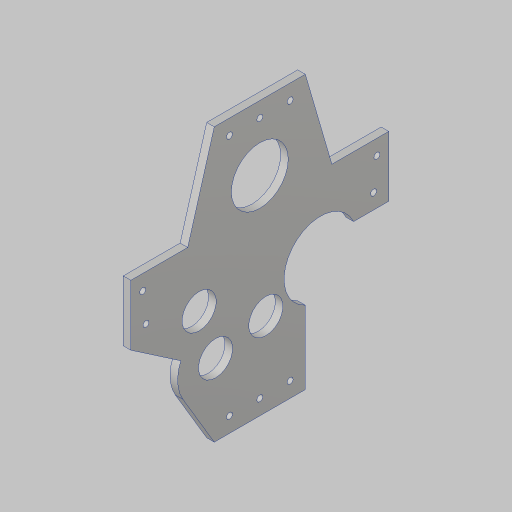
# Autodesk Inventor part: EL2-CGB-003
Saved by Autodesk Inventor 2023.5 (Build 275446000, 446)
## iProperties
Created: 2025-01-19
Part Number: EL2-CGB-003
Material: Aluminum 6061
Document SubType Name: Modeling
Designer: mavericks
Density: 2.7 g/cm^3
Appearance: Aluminum - Flat
Author: mavericks
Autodesk Inventor part; units mm, degrees
ref_plane "YZ Plane" through (0, 0, 0) normal (1, 0, 0) x (0, 1, 0)
ref_plane "XZ Plane" through (0, 0, 0) normal (0, 1, 0) x (-1, 0, 0)
ref_plane "XY Plane" through (0, 0, 0) normal (0, 0, 1) x (1, 0, 0)
sketch "Sketch1" plane through (0, 0, 0) normal (1, 0, 0) x (0, 1, 0)
  line L0 (114.3, 107.95) -> (-114.3, 107.95) construction
  line L1 (-114.3, 107.95) -> (-114.3, 82.55) construction
  line L2 (-114.3, 82.55) -> (114.3, 82.55) construction
  line L3 (114.3, 82.55) -> (114.3, 107.95) construction
  line L4 (-44.45, 128.7526) -> (-69.85, 128.7526) construction
  line L5 (-69.85, 128.7526) -> (-69.85, 79.4258) construction
  line L6 (-69.85, 79.4258) -> (-44.45, 79.4258) construction
  line L7 (-44.45, 79.4258) -> (-44.45, 128.7526) construction
  line L8 (69.85, 128.7526) -> (44.45, 128.7526) construction
  line L9 (44.45, 128.7526) -> (44.45, 79.4258) construction
  line L10 (44.45, 79.4258) -> (69.85, 79.4258) construction
  line L11 (69.85, 79.4258) -> (69.85, 128.7526) construction
  line L12 (44.45, 104.0892) -> (-44.45, 104.0892) construction
  line L13 (0, 0) -> (-27.2932, 0) construction
  line L14 (114.3, -107.95) -> (-114.3, -107.95) construction
  line L15 (-114.3, -107.95) -> (-114.3, -82.55) construction
  line L16 (-114.3, -82.55) -> (114.3, -82.55) construction
  line L17 (114.3, -82.55) -> (114.3, -107.95) construction
  line L18 (-44.45, -128.7526) -> (-69.85, -128.7526) construction
  line L19 (-69.85, -128.7526) -> (-69.85, -79.4258) construction
  line L20 (-69.85, -79.4258) -> (-44.45, -79.4258) construction
  line L21 (-44.45, -79.4258) -> (-44.45, -128.7526) construction
  line L22 (69.85, -128.7526) -> (44.45, -128.7526) construction
  line L23 (44.45, -128.7526) -> (44.45, -79.4258) construction
  line L24 (44.45, -79.4258) -> (69.85, -79.4258) construction
  line L25 (69.85, -79.4258) -> (69.85, -128.7526) construction
  line L26 (44.45, -104.0892) -> (-44.45, -104.0892) construction
  line L27 (114.3, 82.55) -> (88.9, 82.55) construction
  line L28 (88.9, 82.55) -> (88.9, -82.55) construction
  line L29 (88.9, -82.55) -> (114.3, -82.55) construction
  line L30 (114.3, -82.55) -> (114.3, 82.55) construction
  line L31 (-114.3, 82.55) -> (-88.9, 82.55) construction
  line L32 (-88.9, 82.55) -> (-88.9, -82.55) construction
  line L33 (-88.9, -82.55) -> (-114.3, -82.55) construction
  line L34 (-114.3, -82.55) -> (-114.3, 82.55) construction
  point P0 (0, 82.55)
  point P1 (0, 104.0892)
  point P2 (0, -82.55)
  point P3 (0, -104.0892)
  dimension "d0" = 228.6
  dimension "d1" = 25.4
  dimension "d2" = 82.55
  dimension "d3" = 25.4
  dimension "d4" = 49.3268
  dimension "d6" = 88.9
  dimension "d7" = 3.1242
  dimension "d8" = 25.4
  dimension "d9" = 25.4
  constraints: 70 end point, 16 symmetric about line, 12 parallel, 7 horizontal, 5 perpendicular, 4 midpoint, 2 vertical alignment, 1 horizontal alignment, 1 point on line
  measures "d0" distance of L2.end L1.end
  measures "d1" distance of L1.end L0.end
  measures "d2" vertical distance of L13.start L2.end
  measures "d3" distance of L6.end L5.end
  measures "d4" distance of L5.end L4.end
  measures "d6" distance of L4.start L8.end
  measures "d7" distance from line of L2 L6.end
  measures "d8" distance between parallel lines of L28 L30
  measures "d9" distance between parallel lines of L34 L32
sketch "Sketch2" plane through (0, 0, 0) normal (1, 0, 0) x (0, 1, 0)
  line L0 (-114.3, 107.95) -> (-114.3, 82.55) construction
  line L1 (44.45, 104.0892) -> (-44.45, 104.0892) construction
  line L2 (-114.3, 82.55) -> (114.3, 82.55) construction
  line L3 (114.3, 107.95) -> (-114.3, 107.95) construction
  line L4 (44.45, 79.4258) -> (69.85, 79.4258) construction
  line L5 (114.3, 82.55) -> (114.3, 107.95) construction
  line L6 (-69.85, 79.4258) -> (-44.45, 79.4258) construction
  line L7 (-44.45, 79.4258) -> (-44.45, 128.7526) construction
  line L8 (-69.85, 128.7526) -> (-69.85, 79.4258) construction
  line L9 (-44.45, 128.7526) -> (-69.85, 128.7526) construction
  line L10 (88.9, 82.55) -> (88.9, -82.55) construction
  line L11 (114.3, -82.55) -> (114.3, 82.55) construction
  line L12 (-114.3, -82.55) -> (114.3, -82.55) construction
  line L13 (114.3, -107.95) -> (-114.3, -107.95) construction
  line L14 (44.45, -104.0892) -> (-44.45, -104.0892) construction
  line L15 (-114.3, 82.55) -> (-88.9, 82.55) construction
  line L16 (-88.9, 82.55) -> (-88.9, -82.55) construction
  line L17 (-114.3, -82.55) -> (-114.3, 82.55) construction
  line L18 (-69.85, -79.4258) -> (-44.45, -79.4258) construction
  line L19 (-88.9, -82.55) -> (-114.3, -82.55) construction
  line L20 (-44.45, -79.4258) -> (-44.45, -128.7526) construction
  line L21 (-44.45, -128.7526) -> (-69.85, -128.7526) construction
  line L22 (-69.85, -128.7526) -> (-69.85, -79.4258) construction
  line L23 (-114.3, -107.95) -> (-114.3, -82.55) construction
  line L24 (44.45, -79.4258) -> (69.85, -79.4258) construction
  line L25 (44.45, -128.7526) -> (44.45, -79.4258) construction
  line L26 (88.9, -82.55) -> (114.3, -82.55) construction
  line L27 (69.85, -128.7526) -> (44.45, -128.7526) construction
  line L28 (69.85, -79.4258) -> (69.85, -128.7526) construction
  line L29 (114.3, -82.55) -> (114.3, -107.95) construction
  line L30 (69.85, 128.7526) -> (44.45, 128.7526) construction
  line L31 (44.45, 128.7526) -> (44.45, 79.4258) construction
  line L32 (69.85, 79.4258) -> (69.85, 128.7526) construction
  line L33 (114.3, 82.55) -> (88.9, 82.55) construction
  circle A0 centre (-25.4, -50.8) radius 7.62 construction
  circle A1 centre (-44.45, -5.08) radius 41.91 construction
  circle A2 centre (-44.45, -5.08) radius 11.43 construction
  circle A3 centre (-53.975, 37.0363) radius 31.75 construction
  circle A4 centre (-53.975, 37.0363) radius 15.24 construction
  circle A5 centre (-13.0473, 50.8) radius 27.94 construction
  circle A6 centre (-25.4, -50.8) radius 30.48 construction
  circle A7 centre (-25.4, -50.8) radius 10.16 construction
  circle A8 centre (-44.45, -5.08) radius 14.2875
  circle A9 centre (-53.975, 37.0363) radius 14.2875
  circle A10 centre (-13.0473, 50.8) radius 14.2875
  circle A11 centre (-13.0473, 50.8) radius 20.6375 construction
  circle A12 centre (-53.975, 37.0363) radius 20.6375 construction
  circle A13 centre (-44.45, -5.08) radius 20.6375 construction
  circle A14 centre (-25.4, -50.8) radius 17.4625 construction
  circle A15 centre (-25.4, -50.8) radius 25.4 construction
  line L34 (-41.275, -131.9276) -> (-41.275, -76.2508) construction
  line L35 (-41.275, -76.2508) -> (-73.025, -76.2508) construction
  line L36 (-73.025, -76.2508) -> (-73.025, -131.9276) construction
  line L37 (-73.025, -131.9276) -> (-41.275, -131.9276) construction
  line L38 (-114.3, -38.1) -> (-114.3, 38.1)
  line L39 (-114.3, 38.1) -> (-41.275, 38.1) construction
  line L40 (-41.275, 38.1) -> (-41.275, 104.0892) construction
  circle A16 centre (-25.4, -50.8) radius 30.48
  circle A17 centre (59.9086, 0) radius 23.8125
  circle A18 centre (59.9086, 0) radius 33.3375 construction
  line L41 (37.9487, 60.325) -> (114.3, 38.1)
  line L42 (114.3, 38.1) -> (114.3, -38.1)
  line L43 (114.3, -38.1) -> (37.9487, -60.325)
  line L44 (37.9487, -60.325) -> (37.9487, -107.95)
  line L45 (37.9487, -107.95) -> (-12.7, -107.95)
  line L46 (37.9487, 60.325) -> (37.9487, 107.95)
  line L47 (37.9487, 107.95) -> (-12.7, 107.95)
  circle A19 centre (-13.0473, 50.8) radius 20.6375 construction
  circle A20 centre (59.9086, 0) radius 57.277 construction
  line L48 (-12.7, 107.95) -> (-41.275, 66.1357)
  line L49 (-70.2044, 64.325) -> (-114.3, 38.1)
  arc A21 (-41.275, 66.1357) -> (-70.2044, 64.325) centre (-53.975, 37.0363) ccw
  line L50 (-53.1081, -38.1) -> (-114.3, -38.1)
  line L51 (-12.7, -78.5081) -> (-12.7, -107.95)
  point P0 (25.2487, 98.0186)
  point P1 (0, 95.25)
  point P2 (25.2487, -98.0186)
  point P3 (0, -95.25)
  point P4 (-25.4, -95.25)
  point P5 (-25.4, 95.25)
  point P6 (114.3, -95.25)
  point P7 (114.3, 95.25)
  point P8 (0, -82.55)
  point P9 (-101.6, 25.4)
  point P10 (-101.6, 0)
  point P11 (-101.6, -25.4)
  point P12 (-88.9, 0)
  point P13 (-101.6, 82.55)
  point P14 (-25.4, -25.4)
  point P15 (-25.4, -33.3375)
  point P16 (-47.397, -38.1)
  point P17 (-40.523, -42.0688)
  point P18 (-47.397, -63.5)
  point P19 (-40.523, -59.5312)
  point P20 (-25.4, -76.2)
  point P21 (-25.4, -68.2625)
  point P22 (-3.403, -63.5)
  point P23 (-10.277, -59.5313)
  point P24 (-3.403, -38.1)
  point P25 (-10.277, -42.0688)
  point P26 (44.45, 104.0892)
  point P27 (-41.275, -76.8195)
  point P28 (-114.3, 0)
  point P29 (-114.3, 0)
  point P30 (88.9, 0)
  point P31 (101.6, 25.4)
  point P32 (101.6, 0)
  point P33 (101.6, -25.4)
  point P34 (101.6, 82.55)
  point P35 (114.3, 0)
  dimension "d33" = 34.925
  dimension "d34" = 50.8
  dimension "d10" = 15.24
  dimension "d11" = 83.82
  dimension "d12" = 22.86
  dimension "d13" = 63.5
  dimension "d14" = 30.48
  dimension "d15" = 55.88
  dimension "d16" = 60.96
  dimension "d19" = 63.5
  dimension "d23" = 20.32
  dimension "d24" = 28.575
  dimension "d26" = 25.4
  dimension "d27" = 25.4
  dimension "d28" = 25.4
  dimension "d29" = 25.4
  dimension "d30" = 6.35
  dimension "d31" = 6.35
  dimension "d32" = 6.35
  dimension "d37" = 360
  dimension "d41" = 3.175
  dimension "d42" = 76.2
  dimension "d60" = 89.0513
  dimension "d63" = 31.75
  dimension "d64" = 44.45
  dimension "d66" = 34.925
  dimension "d67" = 31.75
  dimension "d68" = 47.625
  dimension "d70" = 9.525
  dimension "d71" = 47.625
  dimension "d73" = 88.9
  dimension "d74" = 12.7
  dimension "d75" = 41.275
  dimension "d76" = 114.554
  dimension "d78" = 9.9314
  dimension "d79" = 9.9314
  dimension "d137" = 12.7
  constraints: 37 end point, 20 centre point, 18 vertical alignment, 14 coincident, 11 horizontal alignment, 11 midpoint, 10 point on line, 8 point on circle, 4 tangent, 3 perpendicular, 2 collinear, 2 equal radius, 2 horizontal, 1 vertical, 20 other
  measures "d10" diameter of A0
  measures "d11" diameter of A1
  measures "d12" diameter of A2
  measures "d13" diameter of A3
  measures "d14" diameter of A4
  measures "d15" diameter of A5
  measures "d16" diameter of A6
  measures "d19" distance from line of L16 A0.centre
  measures "d23" diameter of A7
  measures "d24" diameter of A8
  measures "d26" distance of point (-25.4, 95.25) point (0, 95.25)
  measures "d27" distance of point (25.249, 98.019) point (0, 95.25)
  measures "d28" distance of point (-101.6, 0) point (-101.6, 25.4)
  measures "d29" distance of point (-101.6, 0) point (-101.6, -25.4)
  measures "d30" radial gap between concentric circles of A10 A11
  measures "d31" radial gap between concentric circles of A9 A12
  measures "d32" radial gap between concentric circles of A8 A13
  measures "d41" distance between parallel lines of L20 L34
  measures "d42" distance of L38.start L38.end
  measures "d60" distance from line of L5 point (25.249, 98.019)
  measures "d63" distance from line of L12 A0.centre
  measures "d64" distance from line of L16 A1.centre
  measures "d66" distance from line of L16 A3.centre
  measures "d67" distance from line of L2 A5.centre
  measures "d68" diameter of A17
  measures "d70" radial gap between concentric circles of A17 A18
  measures "d71" distance of L41.start L46.end
  measures "d73" distance of A17.centre A5.centre
  measures "d74" horizontal distance of point (25.249, 98.019) L46.end
  measures "d75" diameter of A19
  measures "d76" diameter of A20
  measures "d78" distance from line of point (25.249, 98.019) L3
  measures "d79" distance from line of L13 point (25.249, -98.019)
  measures "d137" distance from line of L51 point (0, -95.25)
extrude "Extrusion1" add sketch "Sketch2" along normal blind 6.35 contours L38 L49 A21 L48 L47 L46 L41 L42 L43 L44 L45 L51 A16 L50
hole "Mount Holes" at (0, -88.9, 82.55) at (0, -114.3, 107.95) at (0, -69.85, 79.4258) at (0, -44.45, -79.4258) at (0, 44.45, -79.4258) at (0, 69.85, -79.4258) at (0, 44.45, -128.7526) at (0, 44.45, 128.7526) at (0, 25.2487, 98.0186) at (0, 0, 95.25) at (0, 25.2487, -98.0186) at (0, 0, -95.25) at (0, -25.4, -95.25) at (0, -25.4, 95.25) at (0, -101.6, 25.4) at (0, -101.6, 0) at (0, -101.6, -25.4) at (0, 101.6, 25.4) at (0, 101.6, 0) at (0, 101.6, -25.4) direction (1, 0, 0) diameter 5.1054 end through all clearance for "Flat Head Machine Screw (82)" size "#10" standard "Ansi Unified Screw Threads"
sketch "Sketch5" plane through (6.35, 0, 0) normal (1, 0, 0) x (0, 0, -1)
  circle A0 centre (0, 101.6) radius 2.5527 projected
  circle A1 centre (25.4, -101.6) radius 2.5527 projected
  circle A2 centre (-25.4, -101.6) radius 2.5527 projected
  circle A3 centre (98.0186, 25.2487) radius 2.5527 projected
  circle A4 centre (-98.0186, 25.2487) radius 2.5527 projected
  circle A5 centre (-95.25, 0) radius 2.5527 projected
  circle A6 centre (95.25, 0) radius 2.5527 projected
  circle A7 centre (0, -101.6) radius 2.5527 projected
  circle A8 centre (-25.4, 101.6) radius 2.5527 projected
  circle A9 centre (25.4, 101.6) radius 2.5527 projected
  circle A10 centre (5.08, -44.45) radius 14.2875 projected
  circle A11 centre (-37.0363, -53.975) radius 14.2875 projected
  circle A12 centre (-50.8, -13.0473) radius 14.2875 projected
  circle A13 centre (0, 59.9086) radius 23.8125 projected
  line L0 (38.1, -114.3) -> (-38.1, -114.3) projected
  line L1 (-38.1, -114.3) -> (-64.325, -70.2044) projected
  arc A14 (-66.1357, -41.275) -> (-64.325, -70.2044) centre (-37.0363, -53.975) ccw projected
  line L2 (-66.1357, -41.275) -> (-107.95, -12.7) projected
  line L3 (-107.95, -12.7) -> (-107.95, 37.9487) projected
  line L4 (-107.95, 37.9487) -> (-60.325, 37.9487) projected
  line L5 (-60.325, 37.9487) -> (-38.1, 114.3) projected
  line L6 (-38.1, 114.3) -> (38.1, 114.3) projected
  line L7 (38.1, 114.3) -> (60.325, 37.9487) projected
  line L8 (60.325, 37.9487) -> (107.95, 37.9487) projected
  line L9 (107.95, 37.9487) -> (107.95, -12.7) projected
  line L10 (38.1, -53.1081) -> (38.1, -114.3) projected
  line L11 (54.6329, 34.783) -> (33.3349, 107.95) construction
  line L12 (33.3349, 107.95) -> (-33.3349, 107.95) construction
  line L13 (-33.3349, 107.95) -> (-55.5599, 31.5987) construction
  line L14 (-55.5599, 31.5987) -> (-101.6, 31.5987) construction
  line L15 (-101.6, 31.5987) -> (-101.6, -9.3483) construction
  line L16 (-101.6, -9.3483) -> (-57.7691, -39.3014) construction
  arc A15 (-57.7691, -39.3014) -> (-58.8673, -66.9585) centre (-37.0363, -53.975) ccw construction
  line L17 (-58.8673, -66.9585) -> (-34.4884, -107.95) construction
  line L18 (-34.4884, -107.95) -> (31.75, -107.95) construction
  line L19 (31.75, -107.95) -> (31.75, -59.587) construction
  arc A16 (89.8157, -28.4708) -> (31.75, -59.587) centre (50.8, -25.4) ccw construction
  line L20 (89.8157, -28.4708) -> (104.7843, -25.6998) construction
  line L21 (104.7843, -25.6998) -> (104.7843, 34.783) construction
  line L22 (104.7843, 34.783) -> (54.6329, 34.783) construction
  circle A17 centre (0, 59.9086) radius 33.3375 construction
  circle A18 centre (5.08, -44.45) radius 20.6375 construction
  circle A19 centre (-37.0363, -53.975) radius 20.6375 construction
  circle A20 centre (-50.8, -13.0473) radius 20.6375 construction
  circle A21 centre (-95.25, 0) radius 8.9027 construction
  circle A22 centre (-98.0186, 25.2487) radius 8.9027 construction
  circle A23 centre (-95.25, -25.4) radius 8.9027 construction
  circle A24 centre (95.25, -25.4) radius 8.9027 construction
  circle A25 centre (95.25, 0) radius 8.9027 construction
  circle A26 centre (98.0186, 25.2487) radius 8.9027 construction
  circle A27 centre (-25.4, -101.6) radius 8.9027 construction
  circle A28 centre (0, -101.6) radius 8.9027 construction
  circle A29 centre (25.4, -101.6) radius 8.9027 construction
  line L23 (107.95, -12.7) -> (78.5081, -12.7) projected
  arc A30 (78.5081, -12.7) -> (38.1, -53.1081) centre (50.8, -25.4) ccw projected
  point P0 (0, 0)
  dimension "d123" = 6.35
  dimension "d124" = 9.525
  dimension "d125" = 6.35
  dimension "d126" = 6.35
  dimension "d127" = 6.35
  dimension "d128" = 6.35
  dimension "d129" = 6.35
  dimension "d132" = 6.35
  dimension "d133" = 6.35
  dimension "d134" = 6.35
  dimension "d135" = 6.35
  dimension "d136" = 6.35
  constraints: 24 end point, 15 centre point, 4 point on circle, 10 other
  measures "d123" distance between parallel lines of L7 L11
  measures "d124" radial gap between concentric circles of A13 A17
  measures "d125" radial gap between concentric circles of A10 A18
  measures "d126" radial gap between concentric circles of A11 A19
  measures "d127" radial gap between concentric circles of A12 A20
  measures "d128" radial gap between concentric circles of A5 A21
  measures "d129" radial gap between concentric circles of A4 A22
  measures "d132" radial gap between concentric circles of A6 A25
  measures "d133" radial gap between concentric circles of A3 A26
  measures "d134" radial gap between concentric circles of A2 A27
  measures "d135" radial gap between concentric circles of A7 A28
  measures "d136" radial gap between concentric circles of A1 A29
body "Solid1"
